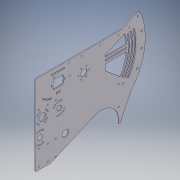
# Autodesk Inventor part: FLY_002_ShooterOuterPlateOutboard
Saved by Autodesk Inventor 2018 (Build 220112000, 112)
## iProperties
Created: 2020-01-28
Part Number: FLY_002_ShooterOuterPlateOutboard
Material: Aluminum 6061, Welded
Document SubType Name: Modeling
Designer: Kevin
Density: 2.7 g/cm^3
Appearance: Weld - Aluminum
Mass: 1432.44 g
Surface Area: 1976.5 cm^2
Volume: 530.532 cm^3
Author: Kevin
Autodesk Inventor part; units mm, degrees
(part 1 of 9)
ref_plane "YZ Plane" through (0, 0, 0) normal (1, 0, 0) x (0, 1, 0)
ref_plane "XZ Plane" through (0, 0, 0) normal (0, 1, 0) x (-1, 0, 0)
ref_plane "XY Plane" through (0, 0, 0) normal (0, 0, 1) x (1, 0, 0)
sketch "Sketch1" plane through (0, 0, 0) normal (1, 0, 0) x (0, 1, 0)
  circle A0 centre (0, 0) radius 7.9375
  line L0 (-391.16, 0) -> (391.16, 0) projected
  line L1 (0, 391.16) -> (0, -391.16) projected
  line L2 (-50.8, 127) -> (76.2, 127)
  line L3 (76.2, 127) -> (76.2, -163.4114)
  line L4 (-50.8, 127) -> (-50.8, -60.5411)
  arc A1 (-163.2681, -194.5753) -> (107.345, -230.2022) centre (0, 0) ccw
  line L5 (0, 0) -> (107.345, -230.2022)
  line L6 (0, 0) -> (-163.2681, -194.5753)
  dimension "d0" = 15.875
  dimension "d1" = 0
  dimension "d2" = 0
  dimension "d5" = 127
  dimension "d6" = 50.8
  dimension "d7" = 127
  dimension "d8" = 254
  dimension "d9" = 25
  dimension "d10" = 40
  constraints: 10 end point, 2 centre point, 2 midpoint, 2 point on circle, 2 point on line, 1 coincident, 1 horizontal, 1 perpendicular, 1 vertical
  measures "d0" diameter of A0
  measures "d1" distance from line of L0 A0.centre
  measures "d2" distance from line of L1 A0.centre
  measures "d5" distance of L2.start L2.end
  measures "d6" distance from line of A0.centre L4
  measures "d7" distance from line of L2 A0.centre
  measures "d8" radius of A1
  measures "d9" angle of L1 L5
  measures "d10" angle of L1 L6
sketch "Sketch2" plane through (0, 0, 0) normal (1, 0, 0) x (0, 1, 0)
  circle A0 centre (0, 0) radius 241.3
  line L0 (0, 0) -> (107.7538, -266.7)
  line L1 (0, 0) -> (287.6452, 0) construction
  line L2 (0, 0) -> (37.5452, -285.1844)
  line L3 (0, 0) -> (287.6452, 0) construction
  line L4 (0, 0) -> (-37.5452, -285.1844)
  line L5 (0, 0) -> (287.6452, 0) construction
  line L6 (0, 0) -> (-114.3759, -263.9279)
  line L7 (0, 0) -> (287.6452, 0) construction
  line L8 (0, 392.3169) -> (0, -398.1012) projected
  circle A1 centre (90.3926, -223.7295) radius 4.7625
  circle A2 centre (31.496, -239.2356) radius 4.7625
  circle A3 centre (-31.496, -239.2356) radius 4.7625
  circle A4 centre (-95.9477, -221.404) radius 4.7625
  dimension "d11" = 482.6
  dimension "d16" = 22
  dimension "d17" = 7.5
  dimension "d18" = 7.5
  dimension "d19" = 23.43
  dimension "d20" = 9.525
  dimension "d21" = 9.525
  dimension "d22" = 9.525
  dimension "d23" = 9.525
  dimension "d24" = 266.7
  constraints: 16 end point, 7 equal length, 5 centre point, 4 horizontal, 4 point on circle, 4 point on line, 1 coincident
  measures "d11" diameter of A0
  measures "d16" angle of L0 L8
  measures "d17" angle of L8 L2
  measures "d18" angle of L8 L4
  measures "d19" angle of L8 L6
  measures "d20" diameter of A1
  measures "d21" diameter of A2
  measures "d22" diameter of A3
  measures "d23" diameter of A4
  measures "d24" vertical distance of L0.start L0.end
sketch "Sketch3" plane through (0, 0, 0) normal (1, 0, 0) x (0, 1, 0)
  circle A0 centre (0, 0) radius 222.25
  line L0 (-391.16, 0) -> (391.16, 0) projected
  line L1 (0, 391.16) -> (0, -391.16) projected
  line L2 (0, 0) -> (100.0571, -247.65)
  line L3 (0, 0) -> (267.0991, 0) construction
  line L4 (0, 0) -> (-160.7443, -213.3148)
  line L5 (0, 0) -> (267.0991, 0) construction
  circle A1 centre (83.2563, -206.0666) radius 3.3147
  circle A2 centre (-133.7534, -177.4967) radius 3.3147
  dimension "d25" = 444.5
  dimension "d26" = 0
  dimension "d27" = 0
  dimension "d30" = 22
  dimension "d31" = 37
  dimension "d32" = 247.65
  dimension "d33" = 6.6294
  dimension "d34" = 6.6294
  constraints: 8 end point, 3 centre point, 3 equal length, 2 horizontal, 2 point on circle, 2 point on line
  measures "d25" diameter of A0
  measures "d26" distance from line of L0 L2.start
  measures "d27" distance from line of L1 L2.start
  measures "d30" angle of L1 L2
  measures "d31" angle of L1 L4
  measures "d32" vertical distance of L2.end L2.start
  measures "d33" diameter of A1
  measures "d34" diameter of A2
extrude "Extrusion1" add sketch "Sketch1" against normal blind 3.175
hole "Hole1" at (0, 90.3926, -223.7295) at (0, 31.496, -239.2356) at (0, -31.496, -239.2356) at (0, -95.9477, -221.404) direction (-1, 0, 0) diameter 6.7564 end through all clearance for "Hex Head Bolt" size "1/4" standard "Ansi Unified Screw Threads"
hole "Hole2" at (0, 0, 0) direction (-1, 0, 0) diameter 15.875 end through all
fillet "Fillet1" radius 12.7 1 edges at (-1.5875, 107.345, -230.2022)
sketch "HS_Inner_Plate" plane through (0, 0, 0) normal (1, 0, 0) x (0, 1, 0)
  circle A0 centre (0, 0) radius 7.9375 projected
  circle A1 centre (0, 0) radius 279.4
  circle A2 centre (0, 0) radius 228.6
  point P0 (0, 0)
  dimension "d52" = 558.8
  dimension "d57" = 457.2
  constraints: 2 centre point, 2 coincident
  measures "d52" diameter of A1
  measures "d57" diameter of A2
sketch "6In_Colson" plane through (0, 0, 0) normal (1, 0, 0) x (0, 1, 0)
  circle A0 centre (0, 0) radius 76.2
  dimension "d53" = 152.4
  constraints: 1 centre point, 1 coincident
  measures "d53" diameter of A0
sketch "Power_Cell" plane through (0, 0, 0) normal (1, 0, 0) x (0, 1, 0)
  circle A0 centre (0, -152.4) radius 88.9
  line L0 (0, 391.16) -> (0, -391.16) projected
  point P0 (0, 0)
  dimension "d54" = 177.8
  dimension "d55" = 152.4
  dimension "d56" = 0
  constraints: 1 centre point
  measures "d54" diameter of A0
  measures "d55" distance of point (0, 0) A0.centre
  measures "d56" distance from line of L0 A0.centre
chamfer "Chamfer1" distance 25.4 angle 45 2 edges at (-1.5875, 76.2, 127) (-1.5875, -50.8, 127)
fillet "Fillet2" radius 50.8 2 edges at (-1.5875, 76.2, -163.4114) (-1.5875, -50.8, -60.5411)
sketch "Sketch8" plane through (0, 0, 0) normal (1, 0, 0) x (0, 0, -1)
  arc A0 (152.4791, -91.4492) -> (177.3458, -12.7) centre (0, 0) ccw
  line L0 (88.9, -38.1) -> (88.9, -12.7)
  line L1 (177.3458, -12.7) -> (88.9, -12.7)
  line L2 (88.9, -38.1) -> (152.4791, -91.4492)
  line L3 (0, -391.16) -> (0, 391.16) projected
  line L4 (-391.16, 0) -> (391.16, 0) projected
  dimension "d72" = 88.9
  dimension "d73" = 40
  dimension "d74" = 177.8
  dimension "d76" = 12.7
  dimension "d77" = 25.4
  constraints: 6 end point, 2 point on circle, 1 centre point, 1 coincident, 1 horizontal
  measures "d72" distance between parallel lines of L3 L0
  measures "d73" angle of L1 L2
  measures "d74" radius of A0
  measures "d76" distance between parallel lines of L4 L1
  measures "d77" distance of L0.start L0.end
extrude "Extrusion3" cut sketch "Sketch8" against normal blind 25.4
sketch "Sketch9" plane through (0, 0, 0) normal (1, 0, 0) x (0, 0, -1)
  line L0 (88.9, 3.175) -> (177.3428, 3.175)
  line L1 (177.3428, 3.175) -> (177.3428, -3.175)
  line L2 (177.3428, -3.175) -> (88.9, -3.175)
  line L3 (88.9, -3.175) -> (88.9, 3.175)
  line L4 (-391.16, 0) -> (391.16, 0) projected
  line L5 (0, -391.16) -> (0, 391.16) projected
  point P0 (0, 0)
  dimension "d80" = 88.4428
  dimension "d81" = 6.35
  dimension "d82" = 3.175
  dimension "d83" = 88.9
  constraints: 8 end point, 2 parallel, 1 horizontal, 1 perpendicular
  measures "d80" distance of L0.start L0.end
  measures "d81" distance of L2.end L0.start
  measures "d82" distance between parallel lines of L4 L2
  measures "d83" distance between parallel lines of L5 L3
extrude "Extrusion4" cut sketch "Sketch9" against normal blind 25.4
sketch "Sketch10" plane through (0, 0, 0) normal (1, 0, 0) x (0, 0, -1)
  line L0 (88.9, 12.7) -> (177.3458, 12.7)
  line L1 (88.9, 12.7) -> (88.9, 19.05)
  line L2 (88.9, 19.05) -> (168.6687, 56.2468)
  arc A0 (177.3458, 12.7) -> (168.6687, 56.2468) centre (0, 0) ccw
  line L3 (0, -391.16) -> (0, 391.16) projected
  line L4 (-391.16, 0) -> (391.16, 0) projected
  dimension "d87" = 6.35
  dimension "d88" = 88.9
  dimension "d89" = 25
  dimension "d90" = 177.8
  dimension "d91" = 12.7
  constraints: 6 end point, 2 point on circle, 1 centre point, 1 coincident, 1 horizontal, 1 vertical
  measures "d87" distance of L0.start L1.end
  measures "d88" distance between parallel lines of L3 L1
  measures "d89" angle of L2 L0
  measures "d90" radius of A0
  measures "d91" distance between parallel lines of L4 L0
extrude "Extrusion5" cut sketch "Sketch10" against normal blind 25.4
fillet "Fillet8" radius 2.921 12 edges at (-1.5875, 19.05, -88.9) (-1.5875, 3.175, -88.9) (-1.5875, 56.2468, -168.6687) (-1.5875, 3.175, -177.3428) (-1.5875, -12.7, -177.3458) (-1.5875, -91.4492, -152.4791) (-1.5875, -38.1, -88.9) (-1.5875, -3.175, -88.9) (-1.5875, 12.7, -88.9) (-1.5875, 12.7, -177.3458) (-1.5875, -12.7, -88.9) (-1.5875, -3.175, -177.3428)
sketch "Sketch11" plane through (0, 0, 0) normal (1, 0, 0) x (0, 0, -1)
  line L0 (25.4, 19.05) -> (82.55, 19.05) construction
  line L1 (82.55, 19.05) -> (82.55, -19.05) construction
  line L2 (82.55, -19.05) -> (25.4, -19.05) construction
  line L3 (25.4, -19.05) -> (25.4, 19.05) construction
  line L4 (-391.16, 0) -> (391.16, 0) projected
  line L5 (0, -391.16) -> (0, 391.16) projected
  point P0 (0, 0)
  dimension "d94" = 38.1
  dimension "d95" = 19.05
  dimension "d96" = 57.15
  dimension "d97" = 25.4
  constraints: 2 other
  measures "d94" distance of L2.end L0.start
  measures "d95" distance between parallel lines of L4 L2
  measures "d96" distance of L0.start L0.end
  measures "d97" distance between parallel lines of L5 L3
extrude "Extrusion6" [suppressed]
sketch "Sketch12" plane through (0, 0, 0) normal (1, 0, 0) x (0, 0, -1)
  line L0 (53.975, 0.7937) -> (82.55, 0.7937)
  line L1 (82.55, 0.7937) -> (82.55, -0.7937)
  line L2 (82.55, -0.7937) -> (53.975, -0.7938)
  line L3 (53.975, -0.7938) -> (53.975, 0.7937)
  line L4 (0, -391.16) -> (0, 391.16) projected
  line L5 (-391.16, 0) -> (391.16, 0) projected
  point P0 (0, 0)
  dimension "d100" = 1.5875
  dimension "d101" = 28.575
  dimension "d102" = 53.975
  dimension "d103" = 0.7937
  constraints: 8 end point, 2 parallel, 1 horizontal, 1 perpendicular
  measures "d100" distance of L2.end L0.start
  measures "d101" distance of L0.start L0.end
  measures "d102" distance between parallel lines of L4 L3
  measures "d103" distance between parallel lines of L5 L2
extrude "Extrusion7" [suppressed]
sketch "Sketch13" plane through (0, 0, 0) normal (1, 0, 0) x (0, 0, -1)
  line L0 (-391.16, 0) -> (391.16, 0) projected
  line L1 (0, -391.16) -> (0, 391.16) projected
  line L2 (0, 0) -> (208.5434, 55.879)
  line L3 (0, 0) -> (228.4441, 0) construction
  line L4 (0, 0) -> (185.0624, -111.1967)
  line L5 (0, 0) -> (215.9, 0) construction
  arc A0 (157.8474, -94.8443) -> (177.8752, 47.6615) centre (0, 0) ccw
  circle A1 centre (0, 0) radius 7.9375 projected
  arc A2 (163.2904, -98.1148) -> (184.0089, 49.305) centre (0, 0) ccw
  arc A3 (168.7334, -101.3852) -> (190.1425, 50.9485) centre (0, 0) ccw
  arc A4 (174.1764, -104.6557) -> (196.2761, 52.592) centre (0, 0) ccw
  arc A5 (179.6194, -107.9262) -> (202.4098, 54.2355) centre (0, 0) ccw
  arc A6 (185.0624, -111.1967) -> (208.5434, 55.879) centre (0, 0) ccw
  dimension "d108" = 0
  dimension "d109" = 0
  dimension "d110" = 15
  dimension "d111" = 31
  dimension "d112" = 184.15
  dimension "d113" = 190.5
  dimension "d114" = 196.85
  dimension "d115" = 203.2
  dimension "d118" = 209.55
  dimension "d119" = 215.9
  constraints: 13 point on circle, 10 point on line, 8 end point, 6 centre point, 4 coincident, 2 horizontal, 1 concentric, 1 midpoint
  measures "d108" distance from line of L0 L2.start
  measures "d109" distance from line of L1 L2.start
  measures "d110" angle of L3 L2
  measures "d111" angle of L4 L5
  measures "d112" radius of A0
  measures "d113" radius of A2
  measures "d114" radius of A3
  measures "d115" radius of A4
  measures "d118" radius of A5
  measures "d119" radius of A6
extrude "Extrusion8" cut sketch "Sketch13" against normal blind 25.4 contours A0 L2 A2 L0 | L0 A2 L4 A0 | A3 L2 A4 L0 | L0 A4 L4 A3 | A5 L2 A6 L0 | L0 A6 L4 A5
fillet "Fillet9" radius 2.54 12 edges at (-1.5875, -111.1967, -185.0624) (-1.5875, -104.6557, -174.1764) (-1.5875, -98.1148, -163.2904) (-1.5875, -107.9262, -179.6194) (-1.5875, -101.3852, -168.7334) (-1.5875, -94.8443, -157.8474) (-1.5875, 55.879, -208.5434) (-1.5875, 52.592, -196.2761) (-1.5875, 49.305, -184.0089) (-1.5875, 54.2355, -202.4098) (-1.5875, 50.9485, -190.1425) (-1.5875, 47.6615, -177.8752)
sketch "Sketch14" plane through (0, 0, 0) normal (1, 0, 0) x (0, 1, 0)
  line L0 (-393.481, 0) -> (405.0857, 0) projected
  line L1 (0, 391.16) -> (0, -391.16) projected
  line L2 (0, 0) -> (-163.2681, -194.5753)
  line L3 (0, 0) -> (281.6971, 0) construction
  line L4 (0, 0) -> (-173.2276, -185.7638)
  line L5 (0, 0) -> (291.0048, 0) construction
  circle A0 centre (0, 0) radius 7.9375 projected
  arc A1 (-173.2276, -185.7638) -> (-163.2681, -194.5753) centre (0, 0) ccw
  arc A2 (-129.9207, -139.3229) -> (-122.451, -145.9315) centre (0, 0) ccw
  dimension "d121" = 0
  dimension "d122" = 0
  dimension "d126" = 254
  dimension "d127" = 190.5
  dimension "d128" = 40
  dimension "d129" = 43
  constraints: 8 end point, 4 point on circle, 2 centre point, 2 horizontal, 2 point on line, 1 coincident
  measures "d121" distance from line of L0 L2.start
  measures "d122" distance from line of L1 L2.start
  measures "d126" radius of A1
  measures "d127" radius of A2
  measures "d128" angle of L2 L1
  measures "d129" angle of L4 L1
extrude "Extrusion9" add sketch "Sketch14" against normal blind 3.175 contours L2 A1 L4 A2
fillet "Fillet3" radius 3.175 1 edges at (-1.5875, -122.451, -145.9315)
chamfer "Chamfer2" distance 3.175 angle 45 1 edges at (-1.5875, -129.9207, -139.3229)
fillet "Fillet4" radius 12.7 1 edges at (-1.5875, -173.2276, -185.7638)
fillet "Fillet5" radius 1.5875 2 edges at (-1.5875, -127.5807, -141.4688) (-1.5875, -132.086, -141.6449)
sketch "Sketch15" plane through (0, 0, 0) normal (1, 0, 0) x (0, 1, 0)
  circle A0 centre (0, 0) radius 200.025
  line L0 (0, 391.16) -> (0, -391.16) projected
  line L1 (-391.16, 0) -> (391.16, 0) projected
  circle A1 centre (0, 0) radius 7.9375 projected
  line L2 (0, 0) -> (-151.085, -204.1796)
  arc A2 (-163.2104, -194.6236) -> (95.0804, -235.5329) centre (0, 0) ccw projected
  line L3 (0, 0) -> (254, 0) construction
  circle A3 centre (-118.9794, -160.7915) radius 1.5875
  circle A4 centre (0, 0) radius 7.9375 projected
  line L4 (0, 0) -> (68.4126, -187.962)
  point P0 (68.4126, -187.962)
  dimension "d137" = 400.05
  dimension "d138" = 0
  dimension "d139" = 0
  dimension "d141" = 3.175
  dimension "d150" = 36.5
  dimension "d553" = 20
  constraints: 6 end point, 4 point on circle, 2 centre point, 2 point on line, 1 equal length, 1 horizontal
  measures "d137" diameter of A0
  measures "d138" distance from line of L0 A0.centre
  measures "d139" distance from line of L1 A0.centre
  measures "d141" diameter of A3
  measures "d150" angle of L0 L2
  measures "d553" angle of L4 L0
hole "Hole3" at (0, -118.9794, -160.7915) at (0, 68.4126, -187.962) direction (-1, 0, 0) diameter 5.1054 end through all clearance for "Flat Head Machine Screw (82)" size "#10" standard "Ansi Unified Screw Threads"
sketch "Sketch16" plane through (0, 0, 0) normal (1, 0, 0) x (0, 0, -1)
  circle A0 centre (160.7915, -118.9794) radius 2.5527 projected
  line L0 (171.9854, -103.3393) -> (170.8967, -102.6851) projected
  arc A1 (170.0112, -99.2275) -> (190.7761, 48.5222) centre (0, 0) ccw projected
  line L1 (192.5803, 51.6017) -> (193.8071, 51.9305) projected
  arc A2 (175.4872, -102.4426) -> (196.9261, 50.1033) centre (0, 0) ccw projected
  arc A3 (159.1231, -92.6879) -> (178.5072, 45.237) centre (0, 0) ccw projected
  line L2 (180.312, 48.3145) -> (181.5388, 48.6432) projected
  arc A4 (164.6013, -95.8992) -> (184.6584, 46.8139) centre (0, 0) ccw projected
  line L3 (161.0985, -96.7977) -> (160.0098, -96.1436) projected
  arc A5 (180.8991, -105.7674) -> (203.0448, 51.8076) centre (0, 0) ccw projected
  line L4 (204.8485, 54.889) -> (206.0753, 55.2177) projected
  arc A6 (186.3731, -108.9857) -> (209.1938, 53.3924) centre (0, 0) ccw projected
  line L5 (182.8723, -109.8807) -> (181.7836, -109.2266) projected
  circle A7 centre (0, 0) radius 7.9375 projected
  circle A8 centre (239.2356, -31.496) radius 3.3782 projected
  circle A9 centre (223.7295, 90.3926) radius 3.3782 projected
  circle A10 centre (239.2356, 31.496) radius 3.3782 projected
  circle A11 centre (221.404, -95.9477) radius 3.3782 projected
  arc A12 (141.6194, -131.4328) -> (142.123, -132.5318) centre (143.2057, -131.3708) ccw projected
  line L6 (142.123, -132.5318) -> (176.2311, -164.3381) projected
  arc A13 (176.2311, -164.3381) -> (194.6236, -163.2104) centre (184.8924, -155.0499) ccw projected
  arc A14 (194.6236, -163.2104) -> (235.5329, 95.0804) centre (0, 0) ccw projected
  arc A15 (235.5329, 95.0804) -> (218.389, 101.8364) centre (223.7562, 90.3263) ccw projected
  line L7 (218.389, 101.8364) -> (173.6183, 80.9596) projected
  arc A16 (152.1493, 76.2) -> (173.6183, 80.9596) centre (152.1493, 127) ccw projected
  line L8 (152.1493, 76.2) -> (-101.6, 76.2) projected
  line L9 (-127, 50.8) -> (-101.6, 76.2) projected
  line L10 (-127, 50.8) -> (-127, -25.4) projected
  line L11 (-101.6, -50.8) -> (-127, -25.4) projected
  line L12 (-101.6, -50.8) -> (42.0514, -50.8) projected
  arc A17 (74.705, -62.6849) -> (42.0514, -50.8) centre (42.0514, -101.6) ccw projected
  line L13 (74.705, -62.6849) -> (143.4787, -120.3929) projected
  arc A18 (143.8351, -124.9069) -> (143.4787, -120.3929) centre (141.4378, -122.8251) ccw projected
  arc A19 (141.8978, -127.1034) -> (143.8351, -124.9069) centre (0, 0) ccw projected
  arc A20 (141.8978, -127.1034) -> (141.494, -128.2246) centre (143.0803, -128.1626) ccw projected
  line L14 (141.6194, -131.4328) -> (141.494, -128.2246) projected
  line L15 (149.831, -89.2272) -> (89.9434, -38.9755) projected
  line L16 (88.9, -36.7379) -> (88.9, -15.621) projected
  line L17 (91.821, -12.7) -> (174.1799, -12.7) projected
  arc A21 (154.2425, -88.4425) -> (177.0893, -15.8819) centre (0, 0) ccw projected
  line L18 (88.9, -0.254) -> (88.9, 0.254) projected
  line L19 (91.821, 3.175) -> (174.4218, 3.175) projected
  line L20 (177.3428, 0.254) -> (177.3428, -0.254) projected
  line L21 (174.4218, -3.175) -> (91.821, -3.175) projected
  arc A22 (177.0893, 15.8819) -> (169.6939, 53.0738) centre (0, 0) ccw projected
  line L22 (174.1799, 12.7) -> (91.821, 12.7) projected
  line L23 (88.9, 15.621) -> (88.9, 17.1891) projected
  line L24 (90.5865, 19.8364) -> (165.6716, 54.8492) projected
  arc A23 (174.1799, 12.7) -> (177.0893, 15.8819) centre (174.1799, 15.621) ccw projected
  arc A24 (88.9, 15.621) -> (91.821, 12.7) centre (91.821, 15.621) ccw projected
  arc A25 (90.5865, 19.8364) -> (88.9, 17.1891) centre (91.821, 17.1891) ccw projected
  arc A26 (169.6939, 53.0738) -> (165.6716, 54.8492) centre (166.9061, 52.2019) ccw projected
  arc A27 (91.821, 3.175) -> (88.9, 0.254) centre (91.821, 0.254) ccw projected
  arc A28 (177.3428, 0.254) -> (174.4218, 3.175) centre (174.4218, 0.254) ccw projected
  arc A29 (174.4218, -3.175) -> (177.3428, -0.254) centre (174.4218, -0.254) ccw projected
  arc A30 (88.9, -0.254) -> (91.821, -3.175) centre (91.821, -0.254) ccw projected
  arc A31 (88.9, -36.7379) -> (89.9434, -38.9755) centre (91.821, -36.7379) ccw projected
  arc A32 (91.821, -12.7) -> (88.9, -15.621) centre (91.821, -15.621) ccw projected
  arc A33 (177.0893, -15.8819) -> (174.1799, -12.7) centre (174.1799, -15.621) ccw projected
  arc A34 (149.831, -89.2272) -> (154.2425, -88.4425) centre (151.7086, -86.9895) ccw projected
  arc A35 (170.0112, -99.2275) -> (170.8967, -102.6851) centre (172.2049, -100.5079) ccw projected
  arc A36 (192.5803, 51.6017) -> (190.7761, 48.5222) centre (193.2377, 49.1483) ccw projected
  arc A37 (196.9261, 50.1033) -> (193.8071, 51.9305) centre (194.4645, 49.477) ccw projected
  arc A38 (171.9854, -103.3393) -> (175.4872, -102.4426) centre (173.2936, -101.1621) ccw projected
  arc A39 (180.312, 48.3145) -> (178.5072, 45.237) centre (180.9694, 45.861) ccw projected
  arc A40 (184.6584, 46.8139) -> (181.5388, 48.6432) centre (182.1962, 46.1897) ccw projected
  arc A41 (161.0985, -96.7977) -> (164.6013, -95.8992) centre (162.4067, -94.6205) ccw projected
  arc A42 (159.1231, -92.6879) -> (160.0098, -96.1436) centre (161.3179, -93.9664) ccw projected
  arc A43 (204.8485, 54.889) -> (203.0448, 51.8076) centre (205.5059, 52.4355) ccw projected
  arc A44 (209.1938, 53.3924) -> (206.0753, 55.2177) centre (206.7327, 52.7643) ccw projected
  arc A45 (182.8723, -109.8807) -> (186.3731, -108.9857) centre (184.1805, -107.7035) ccw projected
  arc A46 (180.8991, -105.7674) -> (181.7836, -109.2266) centre (183.0918, -107.0494) ccw projected
  constraints: 1 coincident
hole "Flywheel Bearing Hole" at (0, 0, 0) direction (-1, 0, 0) diameter 26.67 end through all
sketch "Sketch17" plane through (0, 0, 0) normal (1, 0, 0) x (0, 0, -1)
  circle A0 centre (0, 0) radius 13.335 projected
  circle A1 centre (160.7915, -118.9794) radius 2.5527 projected
  line L0 (171.9854, -103.3393) -> (170.8967, -102.6851) projected
  arc A2 (170.0112, -99.2275) -> (190.7761, 48.5222) centre (0, 0) ccw projected
  line L1 (192.5803, 51.6017) -> (193.8071, 51.9305) projected
  arc A3 (175.4872, -102.4426) -> (196.9261, 50.1033) centre (0, 0) ccw projected
  arc A4 (159.1231, -92.6879) -> (178.5072, 45.237) centre (0, 0) ccw projected
  line L2 (180.312, 48.3145) -> (181.5388, 48.6432) projected
  arc A5 (164.6013, -95.8992) -> (184.6584, 46.8139) centre (0, 0) ccw projected
  line L3 (161.0985, -96.7977) -> (160.0098, -96.1436) projected
  arc A6 (180.8991, -105.7674) -> (203.0448, 51.8076) centre (0, 0) ccw projected
  line L4 (204.8485, 54.889) -> (206.0753, 55.2177) projected
  arc A7 (186.3731, -108.9857) -> (209.1938, 53.3924) centre (0, 0) ccw projected
  line L5 (182.8723, -109.8807) -> (181.7836, -109.2266) projected
  circle A8 centre (239.2356, -31.496) radius 3.3782 projected
  circle A9 centre (223.7295, 90.3926) radius 3.3782 projected
  circle A10 centre (239.2356, 31.496) radius 3.3782 projected
  circle A11 centre (221.404, -95.9477) radius 3.3782 projected
  arc A12 (141.6194, -131.4328) -> (142.123, -132.5318) centre (143.2057, -131.3708) ccw projected
  line L6 (142.123, -132.5318) -> (176.2311, -164.3381) projected
  arc A13 (176.2311, -164.3381) -> (194.6236, -163.2104) centre (184.8924, -155.0499) ccw projected
  arc A14 (194.6236, -163.2104) -> (235.5329, 95.0804) centre (0, 0) ccw projected
  arc A15 (235.5329, 95.0804) -> (218.389, 101.8364) centre (223.7562, 90.3263) ccw projected
  line L7 (218.389, 101.8364) -> (173.6183, 80.9596) projected
  arc A16 (152.1493, 76.2) -> (173.6183, 80.9596) centre (152.1493, 127) ccw projected
  line L8 (152.1493, 76.2) -> (-101.6, 76.2) projected
  line L9 (-127, 50.8) -> (-101.6, 76.2) projected
  line L10 (-127, 50.8) -> (-127, -25.4) projected
  line L11 (-101.6, -50.8) -> (-127, -25.4) projected
  line L12 (-101.6, -50.8) -> (42.0514, -50.8) projected
  arc A17 (74.705, -62.6849) -> (42.0514, -50.8) centre (42.0514, -101.6) ccw projected
  line L13 (74.705, -62.6849) -> (143.4787, -120.3929) projected
  arc A18 (143.8351, -124.9069) -> (143.4787, -120.3929) centre (141.4378, -122.8251) ccw projected
  arc A19 (141.8978, -127.1034) -> (143.8351, -124.9069) centre (0, 0) ccw projected
  arc A20 (141.8978, -127.1034) -> (141.494, -128.2246) centre (143.0803, -128.1626) ccw projected
  line L14 (141.6194, -131.4328) -> (141.494, -128.2246) projected
  line L15 (149.831, -89.2272) -> (89.9434, -38.9755) projected
  line L16 (88.9, -36.7379) -> (88.9, -15.621) projected
  line L17 (91.821, -12.7) -> (174.1799, -12.7) projected
  arc A21 (154.2425, -88.4425) -> (177.0893, -15.8819) centre (0, 0) ccw projected
  line L18 (88.9, -0.254) -> (88.9, 0.254) projected
  line L19 (91.821, 3.175) -> (174.4218, 3.175) projected
  line L20 (177.3428, 0.254) -> (177.3428, -0.254) projected
  line L21 (174.4218, -3.175) -> (91.821, -3.175) projected
  arc A22 (177.0893, 15.8819) -> (169.6939, 53.0738) centre (0, 0) ccw projected
  line L22 (174.1799, 12.7) -> (91.821, 12.7) projected
  line L23 (88.9, 15.621) -> (88.9, 17.1891) projected
  line L24 (90.5865, 19.8364) -> (165.6716, 54.8492) projected
  circle A23 centre (0, 0) radius 14.2875
  circle A24 centre (-84.1126, -94.817) radius 31.75
  line L25 (-136.8951, -14.5284) -> (-96.0159, -31.9839)
  line L26 (-96.0159, -31.9839) -> (-78.5604, 8.8954)
  line L27 (-78.5604, 8.8954) -> (-119.4397, 26.3508)
  line L28 (-119.4397, 26.3508) -> (-136.8951, -14.5284)
  line L29 (-136.8951, -14.5284) -> (-78.5604, 8.8954) construction
  line L30 (-96.0159, -31.9839) -> (-119.4397, 26.3508) construction
  circle A25 centre (-84.1126, -94.817) radius 44.565
  circle A26 centre (0, 0) radius 15.915
  line L31 (-109.9027, -58.4727) -> (-9.2101, 12.9792)
  line L32 (-44.9527, -116.0901) -> (13.9847, -7.597)
  circle A27 centre (0, 0) radius 47.752
  line L33 (-112.8254, 12.2606) -> (-15.2947, 45.2363)
  circle A28 centre (-107.7278, -2.8165) radius 15.9156
  line L34 (-112.0306, -18.1395) -> (-12.91, -45.9738)
  line L35 (-101.8158, -7.1538) -> (-108.528, -10.1051)
  line L36 (-108.528, -10.1051) -> (-114.4399, -5.7678)
  line L37 (-114.4399, -5.7678) -> (-113.6397, 1.5207)
  line L38 (-113.6397, 1.5207) -> (-106.9276, 4.472)
  line L39 (-106.9276, 4.472) -> (-101.0156, 0.1348)
  line L40 (-101.0156, 0.1348) -> (-101.8158, -7.1538)
  circle A29 centre (-107.7278, -2.8165) radius 7.3323
  circle A30 centre (-84.1126, -94.817) radius 9.5631
  circle A31 centre (-107.7278, -2.8165) radius 9.5631
  circle A32 centre (-84.1126, -94.817) radius 25.4
  circle A33 centre (-107.7278, -2.8165) radius 25.4
  line L41 (-84.1126, -94.817) -> (0, 0)
  circle A34 centre (0, 0) radius 50.8
  circle A35 centre (-107.7278, -2.8165) radius 31.4309
  arc A36 (136.2027, -114.2876) -> (161.1415, 75.1415) centre (0, 0) ccw
  line L42 (0, 0) -> (136.2027, -114.2876)
  line L43 (0, 0) -> (129.8014, 0)
  circle A37 centre (42.625, -133.0383) radius 88.9
  circle A38 centre (-86.0916, -204.799) radius 50.8
  line L44 (-82.1889, -38.8068) -> (-89.5385, -28.4495)
  circle A39 centre (-86.0916, -204.799) radius 44.565
  line L45 (-128.6704, -94.0152) -> (-130.6494, -203.9972)
  line L46 (-39.5548, -95.6188) -> (-41.5338, -205.6007)
  line L47 (136.2027, -114.2876) -> (100.1842, -318.5585)
  circle A40 centre (40.4197, -145.5454) radius 88.9
  line L48 (-36.0633, -213.6203) -> (114.0214, -240.0843)
  line L49 (-107.7278, -2.8165) -> (0, 0)
  line L50 (-86.0916, -255.599) -> (-86.0916, -204.799)
  line L51 (136.2027, -114.2876) -> (136.2027, -318.5585)
  line L52 (-60.5854, -2.8165) -> (-107.7278, -2.8165)
  circle A41 centre (12.5242, -303.7486) radius 88.9
  line L53 (-501.4434, -534.4585) -> (248.5176, -534.4585)
  line L54 (-550.7161, -610.6585) -> (328.0098, -610.6585)
  circle A42 centre (-54.61, -445.5585) radius 88.9
  line L55 (-54.61, -359.8335) -> (-16.51, -359.8335)
  line L56 (-16.51, -359.8335) -> (-16.51, -442.3835)
  line L57 (-16.51, -442.3835) -> (-54.61, -442.3835)
  line L58 (-54.61, -442.3835) -> (-54.61, -359.8335)
  line L59 (-54.61, -401.1085) -> (-16.51, -401.1085)
  line L60 (-54.61, -445.5585) -> (-54.61, -356.6585)
  circle A43 centre (-16.51, -356.6585) radius 88.9
  line L61 (-16.51, -356.6585) -> (-16.51, -445.5585)
  arc A44 (-167.6907, -96.0471) -> (-145.5558, -41.5753) centre (-167.732, -64.2971) ccw
  circle A45 centre (-167.732, -64.2971) radius 25.4
  circle A46 centre (-167.732, -64.2971) radius 15.9156
  circle A47 centre (-167.732, -64.2971) radius 9.5631
  line L62 (-181.4932, -72.2932) -> (-99.8528, -212.7951)
  line L63 (-153.9708, -56.301) -> (-72.3304, -196.8029)
  circle A48 centre (-86.0916, -204.799) radius 15.9156
  line L64 (-145.5558, -41.5753) -> (-129.6811, -25.31)
  line L65 (-137.9065, -75.183) -> (-125.9763, -79.5373)
  circle A49 centre (35.0543, -135.2305) radius 88.9
  line L66 (-127, 50.8) -> (-199.482, -21.682)
  line L67 (-199.482, -21.682) -> (-199.482, -255.599)
  line L68 (-199.482, -255.599) -> (-35.2916, -255.599)
  line L69 (-35.2916, -255.599) -> (-35.2916, -50.8)
  line L70 (-101.6, -50.8) -> (42.0514, -50.8) projected
  arc A50 (174.1799, 12.7) -> (177.0893, 15.8819) centre (174.1799, 15.621) ccw projected
  arc A51 (88.9, 15.621) -> (91.821, 12.7) centre (91.821, 15.621) ccw projected
  arc A52 (90.5865, 19.8364) -> (88.9, 17.1891) centre (91.821, 17.1891) ccw projected
  arc A53 (169.6939, 53.0738) -> (165.6716, 54.8492) centre (166.9061, 52.2019) ccw projected
  arc A54 (91.821, 3.175) -> (88.9, 0.254) centre (91.821, 0.254) ccw projected
  arc A55 (177.3428, 0.254) -> (174.4218, 3.175) centre (174.4218, 0.254) ccw projected
  arc A56 (174.4218, -3.175) -> (177.3428, -0.254) centre (174.4218, -0.254) ccw projected
  arc A57 (88.9, -0.254) -> (91.821, -3.175) centre (91.821, -0.254) ccw projected
  arc A58 (88.9, -36.7379) -> (89.9434, -38.9755) centre (91.821, -36.7379) ccw projected
  arc A59 (91.821, -12.7) -> (88.9, -15.621) centre (91.821, -15.621) ccw projected
  arc A60 (177.0893, -15.8819) -> (174.1799, -12.7) centre (174.1799, -15.621) ccw projected
  arc A61 (149.831, -89.2272) -> (154.2425, -88.4425) centre (151.7086, -86.9895) ccw projected
  arc A62 (170.0112, -99.2275) -> (170.8967, -102.6851) centre (172.2049, -100.5079) ccw projected
  arc A63 (192.5803, 51.6017) -> (190.7761, 48.5222) centre (193.2377, 49.1483) ccw projected
  arc A64 (196.9261, 50.1033) -> (193.8071, 51.9305) centre (194.4645, 49.477) ccw projected
  arc A65 (171.9854, -103.3393) -> (175.4872, -102.4426) centre (173.2936, -101.1621) ccw projected
  arc A66 (180.312, 48.3145) -> (178.5072, 45.237) centre (180.9694, 45.861) ccw projected
  arc A67 (184.6584, 46.8139) -> (181.5388, 48.6432) centre (182.1962, 46.1897) ccw projected
  arc A68 (161.0985, -96.7977) -> (164.6013, -95.8992) centre (162.4067, -94.6205) ccw projected
  arc A69 (159.1231, -92.6879) -> (160.0098, -96.1436) centre (161.3179, -93.9664) ccw projected
  arc A70 (204.8485, 54.889) -> (203.0448, 51.8076) centre (205.5059, 52.4355) ccw projected
  arc A71 (209.1938, 53.3924) -> (206.0753, 55.2177) centre (206.7327, 52.7643) ccw projected
  arc A72 (182.8723, -109.8807) -> (186.3731, -108.9857) centre (184.1805, -107.7035) ccw projected
  arc A73 (180.8991, -105.7674) -> (181.7836, -109.2266) centre (183.0918, -107.0494) ccw projected
  point P0 (-35.56, -401.1085)
  dimension "d158" = 28.575
  dimension "d159" = 63.5
  dimension "d160" = 44.45
  dimension "d161" = 31.83
  dimension "d162" = 89.13
  dimension "d163" = 95.504
  dimension "d164" = 31.8313
  dimension "d165" = 12.7
  dimension "d166" = 19.1262
  dimension "d167" = 19.1262
  dimension "d168" = 50.8
  dimension "d169" = 50.8
  dimension "d170" = 107.7646
  dimension "d171" = 126.7485
  dimension "d172" = 101.6
  dimension "d173" = 127
  dimension "d174" = 40
  dimension "d175" = 177.8
  dimension "d176" = 101.6
  dimension "d177" = 12.7
  dimension "d178" = 12.7
  dimension "d179" = 109.9998
  dimension "d180" = 152.4
  dimension "d181" = 330.7405
  dimension "d182" = 25
  dimension "d183" = 10
  dimension "d184" = 47.1424
  dimension "d185" = 89.13
  dimension "d186" = 76.2
  dimension "d187" = 685.8
  dimension "d188" = 82.55
  dimension "d189" = 38.1
  dimension "d190" = 60.3527
  dimension "d191" = 35.56
  dimension "d192" = 215.9
  dimension "d193" = 215.9
  dimension "d194" = 12.7
  dimension "d195" = 22.7282
  dimension "d196" = 162.499
  constraints: 90 end point, 27 point on circle, 27 tangent, 24 centre point, 19 coincident, 9 midpoint, 8 equal radius, 7 horizontal, 7 perpendicular, 7 point on line, 6 line through centre, 5 vertical, 4 parallel, 3 concentric, 2 vertical alignment, 1 collinear, 21 other
  measures "d158" diameter of A23
  measures "d159" diameter of A24
  measures "d160" distance of L26.start L26.end
  measures "d161" diameter of A26
  measures "d162" diameter of A25
  measures "d163" diameter of A27
  measures "d164" diameter of A28
  measures "d165" distance between parallel lines of L39 L36
  measures "d166" diameter of A30
  measures "d167" diameter of A31
  measures "d168" diameter of A32
  measures "d169" diameter of A33
  measures "d170" distance of A23.centre point (-107.728, -2.817)
  measures "d171" distance of point (0, 0) A24.centre
  measures "d172" diameter of A34
  measures "d173" radial gap between concentric circles of A36 A34
  measures "d174" angle of L43 L42
  measures "d175" diameter of A37
  measures "d176" diameter of A38
  measures "d177" distance of L44.start L44.end
  measures "d178" distance of A40.centre A37.centre
  measures "d179" distance of point (-84.113, -94.817) A38.centre
  measures "d180" distance of L48.start L48.end
  measures "d181" vertical distance of L50.start A36.end
  measures "d183" angle of L51 L47
  measures "d184" distance of point (-107.728, -2.817) L52.start
  measures "d185" diameter of A39
  measures "d186" distance between parallel lines of L53 L54
  measures "d187" distance from line of A36.end L54
  measures "d188" distance of L57.end L55.start
  measures "d189" distance of L57.start L57.end
  measures "d190" distance of L61.start A41.centre
  measures "d191" horizontal distance of A34.centre point (-35.56, -401.108)
  measures "d192" distance from line of L53 L51.end
  measures "d193" distance from line of L53 L47.end
  measures "d194" distance of L65.start L65.end
  measures "d195" distance of L64.start L64.end
  measures "d196" distance of A44.centre L50.end
extrude "Extrusion10" add sketch "Sketch17" against normal up to surface (3.175 mm away) contours L41 A25 L12 | L12 L69 A49 A25 L41 | A35 L64 A44 L63 A45 L62 L45 A38 L68 L67 L66 L10 | L10 A33 L28 A35 | A25 A49 L63 L12 | L12 A25 | L31 A25 L65 A44 L64 A35 L11 L12 | L12 A25 L31 | L69 A37 L46 A25 A49 | L28 A33 L10 | L10 L25 A33 L28 | L28 A33 L25 | L25 A33 L10 L11 A35 | A25 A37 A49 | L69 L32 L46 A37 | L69 A40 L46 L32 | L10 A33 L25 | L69 A37 L46 A40 | A49 A38 L63 A25 | A25 L32 A37 A40 L46 A49 | A25 L45 L63 A44 L65 | L46 L32 A37 A25 | A37 A25 L46 | L46 A40 A37 L32 | L46 A37 A40 | L69 A49 A40 L46 A37 | L63 A38 L62 L45 A25 | A25 L63 | A25 A37 L32 | A49 L46 A38 | A38 L46 A39 L63 | A25 L63 L45 | A25 A37 | L50 A39 L46 A38 | A38 L45 A39 L50 | A38 A41 L68 | L46 A40 A37 | L69 A40 A49 | L63 A39 L62 A38 | L46 A49 A40 A38 | L46 A40 A49 | L45 L62 A44 L63 | A44 L62 A45 L63 | L45 L62 A38 | A38 L62 A39 L45 | A38 L48 L69 A41 | A41 L69 L68 | L50 A48 L63 A39 | A39 L62 A48 L50 | L69 A38 A40 | L48 A38 L69 | L63 A48 L62 A39 | L63 A46 L62 A45 | A45 L62 A46 L63 | A48 | A46 | A24 | A30 | A32 | A47 picked at (-136.2053, -9.3163) picked at (-130.9982, 0.9974) picked at (-133.2191, -17.1335) picked at (-127.4263, -18.6412)
sketch "Sketch18" plane through (0, 0, 0) normal (1, 0, 0) x (0, 0, -1)
  arc A0 (177.0893, 15.8819) -> (169.6939, 53.0738) centre (0, 0) ccw projected
  line L0 (174.1799, 12.7) -> (91.821, 12.7) projected
  line L1 (88.9, 15.621) -> (88.9, 17.1891) projected
  line L2 (90.5865, 19.8364) -> (165.6716, 54.8492) projected
  line L3 (88.9, -0.254) -> (88.9, 0.254) projected
  line L4 (91.821, 3.175) -> (174.4218, 3.175) projected
  line L5 (177.3428, 0.254) -> (177.3428, -0.254) projected
  line L6 (174.4218, -3.175) -> (91.821, -3.175) projected
  line L7 (149.831, -89.2272) -> (89.9434, -38.9755) projected
  line L8 (88.9, -36.7379) -> (88.9, -15.621) projected
  line L9 (91.821, -12.7) -> (174.1799, -12.7) projected
  arc A1 (154.2425, -88.4425) -> (177.0893, -15.8819) centre (0, 0) ccw projected
  line L10 (-35.2916, -50.8) -> (42.0514, -50.8) projected
  arc A2 (74.705, -62.6849) -> (42.0514, -50.8) centre (42.0514, -101.6) ccw projected
  line L11 (74.705, -62.6849) -> (143.4787, -120.3929) projected
  arc A3 (143.8351, -124.9069) -> (143.4787, -120.3929) centre (141.4378, -122.8251) ccw projected
  arc A4 (141.8978, -127.1034) -> (143.8351, -124.9069) centre (0, 0) ccw projected
  arc A5 (141.8978, -127.1034) -> (141.494, -128.2246) centre (143.0803, -128.1626) ccw projected
  line L12 (141.6194, -131.4328) -> (141.494, -128.2246) projected
  arc A6 (141.6194, -131.4328) -> (142.123, -132.5318) centre (143.2057, -131.3708) ccw projected
  line L13 (142.123, -132.5318) -> (176.2311, -164.3381) projected
  arc A7 (176.2311, -164.3381) -> (194.6236, -163.2104) centre (184.8924, -155.0499) ccw projected
  arc A8 (194.6236, -163.2104) -> (235.5329, 95.0804) centre (0, 0) ccw projected
  arc A9 (235.5329, 95.0804) -> (218.389, 101.8364) centre (223.7562, 90.3263) ccw projected
  line L14 (218.389, 101.8364) -> (173.6183, 80.9596) projected
  arc A10 (152.1493, 76.2) -> (173.6183, 80.9596) centre (152.1493, 127) ccw projected
  line L15 (152.1493, 76.2) -> (-101.6, 76.2) projected
  line L16 (-101.6, 76.2) -> (-199.482, -21.682) projected
  line L17 (-199.482, -21.682) -> (-199.482, -255.599) projected
  line L18 (-199.482, -255.599) -> (-35.2916, -255.599) projected
  line L19 (-35.2916, -255.599) -> (-35.2916, -50.8) projected
  circle A11 centre (221.404, -95.9477) radius 3.3782 projected
  circle A12 centre (239.2356, 31.496) radius 3.3782 projected
  circle A13 centre (223.7295, 90.3926) radius 3.3782 projected
  circle A14 centre (239.2356, -31.496) radius 3.3782 projected
  arc A15 (180.8991, -105.7674) -> (203.0448, 51.8076) centre (0, 0) ccw projected
  line L20 (204.8485, 54.889) -> (206.0753, 55.2177) projected
  arc A16 (186.3731, -108.9857) -> (209.1938, 53.3924) centre (0, 0) ccw projected
  line L21 (182.8723, -109.8807) -> (181.7836, -109.2266) projected
  arc A17 (159.1231, -92.6879) -> (178.5072, 45.237) centre (0, 0) ccw projected
  line L22 (180.312, 48.3145) -> (181.5388, 48.6432) projected
  arc A18 (164.6013, -95.8992) -> (184.6584, 46.8139) centre (0, 0) ccw projected
  line L23 (161.0985, -96.7977) -> (160.0098, -96.1436) projected
  line L24 (171.9854, -103.3393) -> (170.8967, -102.6851) projected
  arc A19 (170.0112, -99.2275) -> (190.7761, 48.5222) centre (0, 0) ccw projected
  line L25 (192.5803, 51.6017) -> (193.8071, 51.9305) projected
  arc A20 (175.4872, -102.4426) -> (196.9261, 50.1033) centre (0, 0) ccw projected
  circle A21 centre (160.7915, -118.9794) radius 2.5527 projected
  circle A22 centre (0, 0) radius 13.335 projected
  arc A23 (88.9, -36.7379) -> (89.9434, -38.9755) centre (91.821, -36.7379) ccw projected
  arc A24 (91.821, -12.7) -> (88.9, -15.621) centre (91.821, -15.621) ccw projected
  arc A25 (177.0893, -15.8819) -> (174.1799, -12.7) centre (174.1799, -15.621) ccw projected
  arc A26 (149.831, -89.2272) -> (154.2425, -88.4425) centre (151.7086, -86.9895) ccw projected
  arc A27 (91.821, 3.175) -> (88.9, 0.254) centre (91.821, 0.254) ccw projected
  arc A28 (177.3428, 0.254) -> (174.4218, 3.175) centre (174.4218, 0.254) ccw projected
  arc A29 (174.4218, -3.175) -> (177.3428, -0.254) centre (174.4218, -0.254) ccw projected
  arc A30 (88.9, -0.254) -> (91.821, -3.175) centre (91.821, -0.254) ccw projected
  arc A31 (174.1799, 12.7) -> (177.0893, 15.8819) centre (174.1799, 15.621) ccw projected
  arc A32 (88.9, 15.621) -> (91.821, 12.7) centre (91.821, 15.621) ccw projected
  arc A33 (90.5865, 19.8364) -> (88.9, 17.1891) centre (91.821, 17.1891) ccw projected
  arc A34 (169.6939, 53.0738) -> (165.6716, 54.8492) centre (166.9061, 52.2019) ccw projected
  arc A35 (204.8485, 54.889) -> (203.0448, 51.8076) centre (205.5059, 52.4355) ccw projected
  arc A36 (209.1938, 53.3924) -> (206.0753, 55.2177) centre (206.7327, 52.7643) ccw projected
  arc A37 (182.8723, -109.8807) -> (186.3731, -108.9857) centre (184.1805, -107.7035) ccw projected
  arc A38 (180.8991, -105.7674) -> (181.7836, -109.2266) centre (183.0918, -107.0494) ccw projected
  arc A39 (180.312, 48.3145) -> (178.5072, 45.237) centre (180.9694, 45.861) ccw projected
  arc A40 (184.6584, 46.8139) -> (181.5388, 48.6432) centre (182.1962, 46.1897) ccw projected
  arc A41 (161.0985, -96.7977) -> (164.6013, -95.8992) centre (162.4067, -94.6205) ccw projected
  arc A42 (159.1231, -92.6879) -> (160.0098, -96.1436) centre (161.3179, -93.9664) ccw projected
  arc A43 (170.0112, -99.2275) -> (170.8967, -102.6851) centre (172.2049, -100.5079) ccw projected
  arc A44 (192.5803, 51.6017) -> (190.7761, 48.5222) centre (193.2377, 49.1483) ccw projected
  arc A45 (196.9261, 50.1033) -> (193.8071, 51.9305) centre (194.4645, 49.477) ccw projected
  arc A46 (171.9854, -103.3393) -> (175.4872, -102.4426) centre (173.2936, -101.1621) ccw projected
  circle A47 centre (0, 0) radius 14.2875
  circle A48 centre (-101.8395, -75.4579) radius 31.75
  line L26 (-136.6519, 12.4896) -> (-99.0534, -11.2202)
  line L27 (-99.0534, -11.2202) -> (-75.3436, 26.3784)
  line L28 (-75.3436, 26.3784) -> (-112.9422, 50.0881)
  line L29 (-112.9422, 50.0881) -> (-136.6519, 12.4896)
  line L30 (-136.6519, 12.4896) -> (-75.3436, 26.3784) construction
  line L31 (-99.0534, -11.2202) -> (-112.9422, 50.0881) construction
  circle A49 centre (-101.8395, -75.4579) radius 44.565
  circle A50 centre (0, 0) radius 15.915
  line L32 (-119.5903, -34.5807) -> (-6.3391, 14.598)
  line L33 (-67.9013, -104.3411) -> (12.12, -10.3147)
  circle A51 centre (0, 0) radius 47.752
  line L34 (-107.8805, 35.2378) -> (-5.6488, 47.4167)
  circle A52 centre (-105.9978, 19.434) radius 15.9156
  line L35 (-113.3646, 5.3259) -> (-22.1029, -42.3286)
  line L36 (-100.8811, 14.182) -> (-107.9877, 12.3768)
  line L37 (-107.9877, 12.3768) -> (-113.1044, 17.6287)
  line L38 (-113.1044, 17.6287) -> (-111.1145, 24.6859)
  line L39 (-111.1145, 24.6859) -> (-104.0078, 26.4911)
  line L40 (-104.0078, 26.4911) -> (-98.8911, 21.2392)
  line L41 (-98.8911, 21.2392) -> (-100.8811, 14.182)
  circle A53 centre (-105.9978, 19.434) radius 7.3323
  circle A54 centre (-101.8395, -75.4579) radius 9.5631
  circle A55 centre (-105.9978, 19.434) radius 9.5631
  circle A56 centre (-101.8395, -75.4579) radius 25.4
  circle A57 centre (-105.9978, 19.434) radius 25.4
  line L42 (-101.8395, -75.4579) -> (0, 0)
  circle A58 centre (0, 0) radius 50.8
  circle A59 centre (-105.9978, 19.434) radius 31.4309
  arc A60 (136.2027, -114.2876) -> (161.1415, 75.1415) centre (0, 0) ccw
  line L43 (0, 0) -> (136.2027, -114.2876)
  line L44 (0, 0) -> (144.344, 0)
  circle A61 centre (33.8645, -135.5333) radius 88.9
  circle A62 centre (-76.4174, -178.6042) radius 25.4
  line L45 (-88.4199, -21.0451) -> (-93.4785, -9.396)
  circle A63 centre (-76.4174, -178.6042) radius 21.4859
  line L46 (-141.7593, -95.2683) -> (-95.6637, -188.1553)
  line L47 (-57.286, -74.4485) -> (-54.9371, -178.1175)
  line L48 (136.2027, -114.2876) -> (90.5518, -239.7125)
  circle A64 centre (31.6927, -141.5004) radius 88.9
  line L49 (-52.5492, -187.2916) -> (90.6599, -239.4154)
  line L50 (-105.9978, 19.434) -> (0, 0)
  line L51 (-76.4174, -204.0042) -> (-76.4174, -178.6042)
  line L52 (136.2027, -114.2876) -> (136.2027, -239.7125)
  line L53 (-58.8554, 19.434) -> (-105.9978, 19.434)
  circle A65 centre (-17.4502, -276.5193) radius 88.9
  line L54 (-501.4434, -455.6125) -> (248.5176, -455.6125)
  line L55 (-550.7161, -581.025) -> (328.0098, -581.025)
  circle A66 centre (-54.61, -366.7125) radius 88.9
  line L56 (-54.61, -280.9875) -> (-16.51, -280.9875)
  line L57 (-16.51, -280.9875) -> (-16.51, -363.5375)
  line L58 (-16.51, -363.5375) -> (-54.61, -363.5375)
  line L59 (-54.61, -363.5375) -> (-54.61, -280.9875)
  line L60 (-54.61, -322.2625) -> (-16.51, -322.2625)
  line L61 (-54.61, -366.7125) -> (-54.61, -277.8125)
  circle A67 centre (-16.51, -277.8125) radius 88.9
  line L62 (-16.51, -277.8125) -> (-16.51, -366.7125)
  circle A68 centre (-180.2765, -142.3655) radius 31.75
  circle A69 centre (-180.2765, -142.3655) radius 25.4
  circle A70 centre (-180.2765, -142.3655) radius 44.563
  circle A71 centre (-180.2765, -142.3655) radius 9.5631
  line L63 (-194.9575, -184.4408) -> (-91.0984, -220.6795)
  line L64 (-165.5955, -100.2902) -> (-61.7364, -136.5289)
  circle A72 centre (-76.4174, -178.6042) radius 44.563
  line L65 (-167.0299, -113.5109) -> (-119.1112, -9.1307)
  line L66 (-156.1209, -121.7605) -> (-135.7449, -104.3796)
  circle A73 centre (29.8359, -136.4768) radius 88.9
  line L67 (-116.4833, -117.4265) -> (-112.2994, -105.4355)
  circle A74 centre (-76.4174, -178.6042) radius 106.233
  point P0 (-84.1126, -94.817)
  point P1 (-35.56, -322.2625)
  point P2 (-101.7058, -75.4251)
  point P3 (-101.9731, -75.491)
  point P4 (-102.2399, -75.5574)
  point P5 (-102.1066, -75.5241)
  dimension "d595" = 63.5
  dimension "d594" = 28.575
  dimension "d596" = 44.45
  dimension "d597" = 31.83
  dimension "d598" = 89.13
  dimension "d599" = 95.504
  dimension "d600" = 31.8313
  dimension "d601" = 12.7
  dimension "d602" = 19.1262
  dimension "d603" = 19.1262
  dimension "d604" = 50.8
  dimension "d605" = 50.8
  dimension "d606" = 107.7646
  dimension "d607" = 126.7485
  dimension "d608" = 101.6
  dimension "d609" = 127
  dimension "d610" = 40
  dimension "d611" = 177.8
  dimension "d612" = 50.8
  dimension "d613" = 12.7
  dimension "d614" = 6.35
  dimension "d615" = 106.233
  dimension "d616" = 152.4
  dimension "d617" = 279.1458
  dimension "d618" = 25
  dimension "d619" = 20
  dimension "d620" = 47.1424
  dimension "d621" = 42.9717
  dimension "d622" = 125.4125
  dimension "d623" = 656.1665
  dimension "d624" = 82.55
  dimension "d625" = 38.1
  dimension "d626" = 1.5989
  dimension "d627" = 35.56
  dimension "d628" = 215.9
  dimension "d629" = 215.9
  dimension "d630" = 26.7819
  dimension "d631" = 109.9998
  dimension "d632" = 581.025
  dimension "d633" = 455.6125
  dimension "d634" = 12.7
  dimension "d635" = 89.1261
  dimension "d679" = 126.6215
  dimension "d680" = 126.8755
  dimension "d681" = 127.0025
  dimension "d682" = 127.1295
  constraints: 84 end point, 31 point on circle, 24 centre point, 24 tangent, 20 coincident, 9 midpoint, 7 perpendicular, 6 equal radius, 6 horizontal, 6 line through centre, 6 point on line, 4 parallel, 4 vertical, 3 concentric, 2 vertical alignment, 26 other
  measures "d594" diameter of A47
  measures "d596" distance of L26.end L30.end
  measures "d597" diameter of A50
  measures "d598" diameter of A49
  measures "d599" diameter of A51
  measures "d600" diameter of A52
  measures "d601" distance between parallel lines of L40 L37
  measures "d602" diameter of A54
  measures "d603" diameter of A55
  measures "d604" diameter of A56
  measures "d605" diameter of A57
  measures "d606" distance of A47.centre point (-105.998, 19.434)
  measures "d607" distance of point (0, 0) point (-101.84, -75.458)
  measures "d608" diameter of A58
  measures "d609" radial gap between concentric circles of A60 A58
  measures "d610" angle of L44 L43
  measures "d611" diameter of A61
  measures "d612" diameter of A62
  measures "d613" distance of L45.start L45.end
  measures "d614" distance of A64.centre A61.centre
  measures "d615" distance of A74.start A62.centre
  measures "d616" distance of L49.start L49.end
  measures "d617" vertical distance of L51.start A60.end
  measures "d619" angle of L52 L48
  measures "d620" distance of point (-105.998, 19.434) L53.start
  measures "d621" diameter of A63
  measures "d622" distance between parallel lines of L54 L55
  measures "d623" distance from line of A60.end L55
  measures "d624" distance of L58.end L56.start
  measures "d625" distance of L58.start L58.end
  measures "d626" distance of L62.start A65.centre
  measures "d627" horizontal distance of A58.centre point (-35.56, -322.262)
  measures "d628" distance from line of L54 L52.end
  measures "d629" distance from line of L54 L48.end
  measures "d630" distance of L66.start L66.end
  measures "d631" distance of A68.centre L51.end
  measures "d632" distance from line of L55 point (0, 0)
  measures "d633" distance from line of L54 L43.start
  measures "d634" distance of L67.start L67.end
  measures "d635" diameter of A70
  measures "d679" distance of L42.end A74.end
  measures "d680" distance of point (0, 0) point (-101.973, -75.491)
  measures "d681" distance of A0.centre point (-102.107, -75.524)
  measures "d682" distance of L42.end point (-102.24, -75.557)
hole "Hole5" at (0, -75.5574, 102.2399) at (0, -75.5241, 102.1066) at (0, -75.491, 101.9731) at (0, -75.4579, 101.8395) at (0, -75.4251, 101.7058) direction (-1, 0, 0) diameter 19.1262 end through all